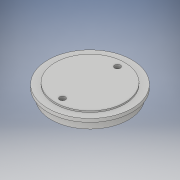
# Autodesk Inventor part: 2016.06.09 Blank Adapter
Saved by Autodesk Inventor 2017 (Build 210142000, 142)
## iProperties
Created: 2016-06-09
Part Number: 2016.06.09 Blank Adapter
Material: Generic
Document SubType Name: Modeling
Designer: Darien Morrow
Density: 1 g/cm^3
Appearance: Default
Author: Darien Morrow
Autodesk Inventor part; units mm, degrees
ref_plane "YZ Plane" through (0, 0, 0) normal (1, 0, 0) x (0, 1, 0)
ref_plane "XZ Plane" through (0, 0, 0) normal (0, 1, 0) x (-1, 0, 0)
ref_plane "XY Plane" through (0, 0, 0) normal (0, 0, 1) x (1, 0, 0)
sketch "Sketch1" plane through (0, 0, 0) normal (0, 0, 1) x (1, 0, 0)
  line L0 (17.5514, 0) -> (46.0756, 0)
  line L1 (46.0756, 0) -> (46.0756, 12.7)
  line L2 (46.0756, 12.7) -> (0, 12.7)
  line L3 (0, 12.7) -> (0, 0)
  line L4 (17.5514, 12.7) -> (17.5514, 0)
  line L5 (46.0756, 8.9662) -> (42.3672, 8.9662)
  line L6 (42.3672, 7.747) -> (42.3672, 0)
  line L7 (46.0756, 7.747) -> (42.3672, 7.747)
  line L8 (46.0756, 8.9662) -> (42.3672, 7.747)
  line L9 (0, 11.1252) -> (0, 12.7)
  line L10 (17.5514, 0) -> (23.85, 0)
  line L11 (0, -2.5) -> (0, 0)
  line L12 (0, 12.7) -> (38.0365, 12.7)
  line L13 (38.0365, 12.7) -> (38.0365, 14.2748)
  line L14 (38.0365, 14.2748) -> (0, 14.2748)
  line L15 (0, 14.2748) -> (0, 12.7)
  line L16 (17.5514, 12.7) -> (17.5514, 14.2748)
  line L17 (0, 0) -> (17.5514, 0)
  dimension "d1" = 12.7
  dimension "d3" = 3.7338
  dimension "d5" = 4.953
  dimension "d8" = 17.5514
  dimension "d9" = 42.3672
  dimension "d10" = 46.0756
  dimension "d11" = 1.5748
  dimension "d12" = 38.0365
  constraints: 36 end point, 7 perpendicular, 7 point on line, 4 horizontal, 4 parallel
  measures "d1" distance of L2.end L3.end
  measures "d3" distance between parallel lines of L5 L2
  measures "d5" distance between parallel lines of L7 L2
  measures "d8" distance between parallel lines of L4 L3
  measures "d9" distance between parallel lines of L6 L3
  measures "d10" distance between parallel lines of L1 L3
  measures "d11" distance between parallel lines of L2 L14
  measures "d12" distance between parallel lines of L13 L15
revolve "Revolution1" add sketch "Sketch1" angle 360 about axis through (0, 12.7, 0) along (0, -1, 0) contours L4 L2 L1 L8 L6 L0 | L17 L3 L2 L4 | L16 L14 L13 L2 | L2 L15 L14 L16
sketch "Sketch2" plane through (0, 14.2748, 0) normal (0, 1, 0) x (1, 0, 0)
  circle A0 centre (0, 0) radius 30.1752
  point P0 (0, 30.1752)
  point P1 (0, -30.1752)
  dimension "d14" = 60.3504
  constraints: 2 point on circle, 1 centre point, 1 coincident
  measures "d14" diameter of A0
hole "Hole1" at (0, 14.2748, -30.1752) at (0, 14.2748, 30.1752) direction (0, -1, 0) diameter 6.35 depth 10.16
body "Solid1"
